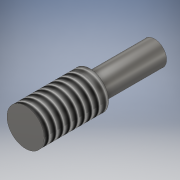
# Autodesk Inventor part: VS-010 (SET SCREW)
Saved by Autodesk Inventor 2017 SP1 (Build 210196100, 196)
## iProperties
Created: 2016-12-07
Part Number: VS-010 (SET SCREW)
Material: Steel, Carbon
Document SubType Name: Modeling
Designer: OCCC
Density: 7.85 g/cm^3
Appearance: Semi-Polished
Author: OCCC
Autodesk Inventor part; units mm, degrees
ref_plane "YZ Plane" through (0, 0, 0) normal (1, 0, 0) x (0, 1, 0)
ref_plane "XZ Plane" through (0, 0, 0) normal (0, 1, 0) x (-1, 0, 0)
ref_plane "XY Plane" through (0, 0, 0) normal (0, 0, 1) x (1, 0, 0)
sketch "Sketch1" plane through (0, 0, 0) normal (0, 0, 1) x (1, 0, 0)
  circle A0 centre (0, 0) radius 2.7432
  dimension "d0" = 5.4864
  constraints: 1 centre point, 1 coincident
  measures "d0" diameter of A0
extrude "Extrusion1" add sketch "Sketch1" against normal blind 9.525
sketch "Sketch2" plane through (0, 0, -9.525) normal (0, 0, -1) x (-1, 0, 0)
  circle A0 centre (0, 0) radius 1.7907
  dimension "d3" = 3.5814
  constraints: 1 centre point, 1 coincident
  measures "d3" diameter of A0
extrude "Extrusion2" add sketch "Sketch2" along normal blind 9.525
thread "Thread1" size "12-24 UNC" class "2A" standard "ANSI Unified Screw Threads" length 9.525 offset 1.1906
thread "Thread2" size "12-24 UNC" class "2A" standard "ANSI Unified Screw Threads" full length
body "Solid1"
